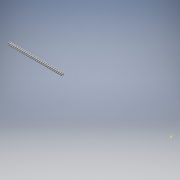
# Autodesk Inventor part: 40401m
Saved by Autodesk Inventor 2019 (Build 230136000, 136)
## iProperties
Company: TraceParts S.A.
Created: 2018-05-03
Part Number: 40401m
Checked By: TraceParts S.A.
Material: Aluminum 6061
Catalog Web Link: www.traceparts.com
Document SubType Name: Modeling
Designer: TraceParts
Density: 2.7 g/cm^3
Appearance: Aluminum - Dark
SUPPLIER_NAME: RS Components
SUPPLIER: Bosch Rexroth
RS_STOCK_NUMBER: 4597211
REVISION: A
DESIGN: Bosch Rexroth Aluminium Strut Profile, 10mm Groove , 3000mm L, 40 x 40mm strut profile
REFERENCE: 3842993120/3000
TIMESTAMP: 30/06/2015 16:02
TraceParts.PartVersion: 1.1.3
TraceParts.PartStatus: Published
TRACEPARTS: TRACEPARTS
TraceParts.InstanceId: 10-20072015-123890AZAWWE1HC2GQYC8QBJ8WTJ7U2
TraceParts.PartLanguage: en
TraceParts.PartTitle: Bosch Rexroth Aluminium Strut Profile, 10mm Groove , 3000mm L, 40 x 40mm strut profile
TraceParts.PartNumber: 10-20072015-123890
TraceParts.ClassPath: RS_COMPONENTS:10-20072015-123890
Author: TraceParts
Autodesk Inventor part; units mm, degrees
ref_plane "YZ Plane" through (0, 0, 0) normal (1, 0, 0) x (0, 1, 0)
ref_plane "XZ Plane" through (0, 0, 0) normal (0, 1, 0) x (-1, 0, 0)
ref_plane "XY Plane" through (0, 0, 0) normal (0, 0, 1) x (1, 0, 0)
ref_plane "Work Plane1" through (3000, -6.0858, -7.5) normal (1, 0, 0) x (0, 0, -1)
sketch "Sketch1" plane through (3000, -6.0858, -7.5) normal (1, 0, 0) x (0, 0, -1)
  line L0 (0, 0) -> (3.9642, -3.9642) projected
  line L1 (0, 12.1716) -> (0, 0) projected
  line L2 (3.9642, 16.1358) -> (0, 12.1716) projected
  line L3 (6.5, 16.1358) -> (3.9642, 16.1358) projected
  line L4 (6.5, 11.0858) -> (6.5, 16.1358) projected
  line L5 (11, 11.0858) -> (6.5, 11.0858) projected
  line L6 (11, 11.8858) -> (11, 11.0858) projected
  line L7 (12.5, 11.8858) -> (11, 11.8858) projected
  line L8 (12.5, 23.0858) -> (12.5, 11.8858) projected
  arc A0 (12.5, 23.0858) -> (9.5, 26.0858) centre (9.5, 23.0858) ccw projected
  line L9 (-1.7, 26.0858) -> (9.5, 26.0858) projected
  line L10 (-1.7, 24.5858) -> (-1.7, 26.0858) projected
  line L11 (-2.5, 24.5858) -> (-1.7, 24.5858) projected
  line L12 (-2.5, 20.0858) -> (-2.5, 24.5858) projected
  line L13 (2.55, 20.0858) -> (-2.5, 20.0858) projected
  line L14 (2.55, 17.55) -> (2.55, 20.0858) projected
  line L15 (-1.4142, 13.5858) -> (2.55, 17.55) projected
  line L16 (-13.5858, 13.5858) -> (-1.4142, 13.5858) projected
  line L17 (-17.55, 17.55) -> (-13.5858, 13.5858) projected
  line L18 (-17.55, 20.0858) -> (-17.55, 17.55) projected
  line L19 (-12.5, 20.0858) -> (-17.55, 20.0858) projected
  line L20 (-12.5, 24.5858) -> (-12.5, 20.0858) projected
  line L21 (-13.3, 24.5858) -> (-12.5, 24.5858) projected
  line L22 (-13.3, 26.0858) -> (-13.3, 24.5858) projected
  line L23 (-24.5, 26.0858) -> (-13.3, 26.0858) projected
  arc A1 (-24.5, 26.0858) -> (-27.5, 23.0858) centre (-24.5, 23.0858) ccw projected
  line L24 (-27.5, 11.8858) -> (-27.5, 23.0858) projected
  line L25 (-26, 11.8858) -> (-27.5, 11.8858) projected
  line L26 (-26, 11.0858) -> (-26, 11.8858) projected
  line L27 (-21.5, 11.0858) -> (-26, 11.0858) projected
  line L28 (-21.5, 16.1358) -> (-21.5, 11.0858) projected
  line L29 (-18.9642, 16.1358) -> (-21.5, 16.1358) projected
  line L30 (-15, 12.1716) -> (-18.9642, 16.1358) projected
  line L31 (-15, 0) -> (-15, 12.1716) projected
  line L32 (-18.9642, -3.9642) -> (-15, 0) projected
  line L33 (-21.5, -3.9642) -> (-18.9642, -3.9642) projected
  line L34 (-21.5, 1.0858) -> (-21.5, -3.9642) projected
  line L35 (-26, 1.0858) -> (-21.5, 1.0858) projected
  line L36 (-26, 0.2858) -> (-26, 1.0858) projected
  line L37 (-27.5, 0.2858) -> (-26, 0.2858) projected
  line L38 (-27.5, -10.9142) -> (-27.5, 0.2858) projected
  arc A2 (-27.5, -10.9142) -> (-24.5, -13.9142) centre (-24.5, -10.9142) ccw projected
  line L39 (-13.3, -13.9142) -> (-24.5, -13.9142) projected
  line L40 (-13.3, -12.4142) -> (-13.3, -13.9142) projected
  line L41 (-12.5, -12.4142) -> (-13.3, -12.4142) projected
  line L42 (-12.5, -7.9142) -> (-12.5, -12.4142) projected
  line L43 (-17.55, -7.9142) -> (-12.5, -7.9142) projected
  line L44 (-17.55, -5.3784) -> (-17.55, -7.9142) projected
  line L45 (-13.5858, -1.4142) -> (-17.55, -5.3784) projected
  line L46 (-1.4142, -1.4142) -> (-13.5858, -1.4142) projected
  line L47 (2.55, -5.3784) -> (-1.4142, -1.4142) projected
  line L48 (2.55, -7.9142) -> (2.55, -5.3784) projected
  line L49 (-2.5, -7.9142) -> (2.55, -7.9142) projected
  line L50 (-2.5, -12.4142) -> (-2.5, -7.9142) projected
  line L51 (-1.7, -12.4142) -> (-2.5, -12.4142) projected
  line L52 (-1.7, -13.9142) -> (-1.7, -12.4142) projected
  line L53 (9.5, -13.9142) -> (-1.7, -13.9142) projected
  arc A3 (9.5, -13.9142) -> (12.5, -10.9142) centre (9.5, -10.9142) ccw projected
  line L54 (12.5, 0.2858) -> (12.5, -10.9142) projected
  line L55 (11, 0.2858) -> (12.5, 0.2858) projected
  line L56 (11, 1.0858) -> (11, 0.2858) projected
  line L57 (6.5, 1.0858) -> (11, 1.0858) projected
  line L58 (6.5, -3.9642) -> (6.5, 1.0858) projected
  line L59 (3.9642, -3.9642) -> (6.5, -3.9642) projected
  line L60 (8, -1.9142) -> (11, -1.9142) projected
  line L61 (11, -1.9142) -> (11, -8.4142) projected
  line L62 (11, -8.4142) -> (9.75, -8.4142) projected
  arc A4 (7, -11.1642) -> (9.75, -8.4142) centre (7, -8.4142) ccw projected
  line L63 (7, -11.1642) -> (7, -12.4142) projected
  line L64 (7, -12.4142) -> (0.5, -12.4142) projected
  line L65 (0.5, -12.4142) -> (0.5, -9.4142) projected
  line L66 (0.5, -9.4142) -> (4.25, -9.4142) projected
  line L67 (4.25, -9.4142) -> (4.25, -8.4142) projected
  arc A5 (7, -5.6642) -> (4.25, -8.4142) centre (7, -8.4142) ccw projected
  line L68 (7, -5.6642) -> (8, -5.6642) projected
  line L69 (8, -5.6642) -> (8, -1.9142) projected
  line L70 (0.5, 21.5858) -> (0.5, 24.5858) projected
  line L71 (0.5, 24.5858) -> (7, 24.5858) projected
  line L72 (7, 24.5858) -> (7, 23.3358) projected
  arc A6 (9.75, 20.5858) -> (7, 23.3358) centre (7, 20.5858) ccw projected
  line L73 (9.75, 20.5858) -> (11, 20.5858) projected
  line L74 (11, 20.5858) -> (11, 14.0858) projected
  line L75 (11, 14.0858) -> (8, 14.0858) projected
  line L76 (8, 14.0858) -> (8, 17.8358) projected
  line L77 (8, 17.8358) -> (7, 17.8358) projected
  arc A7 (4.25, 20.5858) -> (7, 17.8358) centre (7, 20.5858) ccw projected
  line L78 (4.25, 20.5858) -> (4.25, 21.5858) projected
  line L79 (4.25, 21.5858) -> (0.5, 21.5858) projected
  line L80 (-23, 14.0858) -> (-26, 14.0858) projected
  line L81 (-26, 14.0858) -> (-26, 20.5858) projected
  line L82 (-26, 20.5858) -> (-24.75, 20.5858) projected
  arc A8 (-22, 23.3358) -> (-24.75, 20.5858) centre (-22, 20.5858) ccw projected
  line L83 (-22, 23.3358) -> (-22, 24.5858) projected
  line L84 (-22, 24.5858) -> (-15.5, 24.5858) projected
  line L85 (-15.5, 24.5858) -> (-15.5, 21.5858) projected
  line L86 (-15.5, 21.5858) -> (-19.25, 21.5858) projected
  line L87 (-19.25, 21.5858) -> (-19.25, 20.5858) projected
  arc A9 (-22, 17.8358) -> (-19.25, 20.5858) centre (-22, 20.5858) ccw projected
  line L88 (-22, 17.8358) -> (-23, 17.8358) projected
  line L89 (-23, 17.8358) -> (-23, 14.0858) projected
  line L90 (-15.5, -9.4142) -> (-15.5, -12.4142) projected
  line L91 (-15.5, -12.4142) -> (-22, -12.4142) projected
  line L92 (-22, -12.4142) -> (-22, -11.1642) projected
  arc A10 (-24.75, -8.4142) -> (-22, -11.1642) centre (-22, -8.4142) ccw projected
  line L93 (-24.75, -8.4142) -> (-26, -8.4142) projected
  line L94 (-26, -8.4142) -> (-26, -1.9142) projected
  line L95 (-26, -1.9142) -> (-23, -1.9142) projected
  line L96 (-23, -1.9142) -> (-23, -5.6642) projected
  line L97 (-23, -5.6642) -> (-22, -5.6642) projected
  arc A11 (-19.25, -8.4142) -> (-22, -5.6642) centre (-22, -8.4142) ccw projected
  line L98 (-19.25, -8.4142) -> (-19.25, -9.4142) projected
  line L99 (-19.25, -9.4142) -> (-15.5, -9.4142) projected
  line L100 (-9.4937, 1.5005) -> (-9.761, 0.8858) projected
  line L101 (-9.761, 0.8858) -> (-12.7, 0.8858) projected
  line L102 (-12.7, 0.8858) -> (-12.7, 3.8248) projected
  line L103 (-12.7, 3.8248) -> (-12.0853, 4.092) projected
  arc A12 (-12.0853, 8.0795) -> (-12.0853, 4.092) centre (-7.5, 6.0858) ccw projected
  line L104 (-12.0853, 8.0795) -> (-12.7, 8.3468) projected
  line L105 (-12.7, 8.3468) -> (-12.7, 11.2858) projected
  line L106 (-12.7, 11.2858) -> (-9.761, 11.2858) projected
  line L107 (-9.761, 11.2858) -> (-9.4937, 10.6711) projected
  arc A13 (-5.5063, 10.6711) -> (-9.4937, 10.6711) centre (-7.5, 6.0858) ccw projected
  line L108 (-5.5063, 10.6711) -> (-5.239, 11.2858) projected
  line L109 (-5.239, 11.2858) -> (-2.3, 11.2858) projected
  line L110 (-2.3, 11.2858) -> (-2.3, 8.3468) projected
  line L111 (-2.3, 8.3468) -> (-2.9147, 8.0795) projected
  arc A14 (-2.9147, 4.092) -> (-2.9147, 8.0795) centre (-7.5, 6.0858) ccw projected
  line L112 (-2.9147, 4.092) -> (-2.3, 3.8248) projected
  line L113 (-2.3, 3.8248) -> (-2.3, 0.8858) projected
  line L114 (-2.3, 0.8858) -> (-5.239, 0.8858) projected
  line L115 (-5.239, 0.8858) -> (-5.5063, 1.5005) projected
  arc A15 (-9.4937, 1.5005) -> (-5.5063, 1.5005) centre (-7.5, 6.0858) ccw projected
  point P0 (-7.5, 6.0858)
ref_plane "Work Plane2" through (0, -6.0858, -7.5) normal (-1, 0, 0) x (0, 0, 1)
sketch "Sketch2" plane through (0, -6.0858, -7.5) normal (-1, 0, 0) x (0, 0, 1)
  line L0 (0, 12.1716) -> (0, 0) projected
  line L1 (0, 0) -> (-3.9642, -3.9642) projected
  line L2 (-3.9642, -3.9642) -> (-6.5, -3.9642) projected
  line L3 (-6.5, -3.9642) -> (-6.5, 1.0858) projected
  line L4 (-6.5, 1.0858) -> (-11, 1.0858) projected
  line L5 (-11, 1.0858) -> (-11, 0.2858) projected
  line L6 (-11, 0.2858) -> (-12.5, 0.2858) projected
  line L7 (-12.5, 0.2858) -> (-12.5, -10.9142) projected
  arc A0 (-12.5, -10.9142) -> (-9.5, -13.9142) centre (-9.5, -10.9142) ccw projected
  line L8 (-9.5, -13.9142) -> (1.7, -13.9142) projected
  line L9 (1.7, -13.9142) -> (1.7, -12.4142) projected
  line L10 (1.7, -12.4142) -> (2.5, -12.4142) projected
  line L11 (2.5, -12.4142) -> (2.5, -7.9142) projected
  line L12 (2.5, -7.9142) -> (-2.55, -7.9142) projected
  line L13 (-2.55, -7.9142) -> (-2.55, -5.3784) projected
  line L14 (-2.55, -5.3784) -> (1.4142, -1.4142) projected
  line L15 (1.4142, -1.4142) -> (13.5858, -1.4142) projected
  line L16 (13.5858, -1.4142) -> (17.55, -5.3784) projected
  line L17 (17.55, -5.3784) -> (17.55, -7.9142) projected
  line L18 (17.55, -7.9142) -> (12.5, -7.9142) projected
  line L19 (12.5, -7.9142) -> (12.5, -12.4142) projected
  line L20 (12.5, -12.4142) -> (13.3, -12.4142) projected
  line L21 (13.3, -12.4142) -> (13.3, -13.9142) projected
  line L22 (13.3, -13.9142) -> (24.5, -13.9142) projected
  arc A1 (24.5, -13.9142) -> (27.5, -10.9142) centre (24.5, -10.9142) ccw projected
  line L23 (27.5, -10.9142) -> (27.5, 0.2858) projected
  line L24 (27.5, 0.2858) -> (26, 0.2858) projected
  line L25 (26, 0.2858) -> (26, 1.0858) projected
  line L26 (26, 1.0858) -> (21.5, 1.0858) projected
  line L27 (21.5, 1.0858) -> (21.5, -3.9642) projected
  line L28 (21.5, -3.9642) -> (18.9642, -3.9642) projected
  line L29 (18.9642, -3.9642) -> (15, 0) projected
  line L30 (15, 0) -> (15, 12.1716) projected
  line L31 (15, 12.1716) -> (18.9642, 16.1358) projected
  line L32 (18.9642, 16.1358) -> (21.5, 16.1358) projected
  line L33 (21.5, 16.1358) -> (21.5, 11.0858) projected
  line L34 (21.5, 11.0858) -> (26, 11.0858) projected
  line L35 (26, 11.0858) -> (26, 11.8858) projected
  line L36 (26, 11.8858) -> (27.5, 11.8858) projected
  line L37 (27.5, 11.8858) -> (27.5, 23.0858) projected
  arc A2 (27.5, 23.0858) -> (24.5, 26.0858) centre (24.5, 23.0858) ccw projected
  line L38 (24.5, 26.0858) -> (13.3, 26.0858) projected
  line L39 (13.3, 26.0858) -> (13.3, 24.5858) projected
  line L40 (13.3, 24.5858) -> (12.5, 24.5858) projected
  line L41 (12.5, 24.5858) -> (12.5, 20.0858) projected
  line L42 (12.5, 20.0858) -> (17.55, 20.0858) projected
  line L43 (17.55, 20.0858) -> (17.55, 17.55) projected
  line L44 (17.55, 17.55) -> (13.5858, 13.5858) projected
  line L45 (13.5858, 13.5858) -> (1.4142, 13.5858) projected
  line L46 (1.4142, 13.5858) -> (-2.55, 17.55) projected
  line L47 (-2.55, 17.55) -> (-2.55, 20.0858) projected
  line L48 (-2.55, 20.0858) -> (2.5, 20.0858) projected
  line L49 (2.5, 20.0858) -> (2.5, 24.5858) projected
  line L50 (2.5, 24.5858) -> (1.7, 24.5858) projected
  line L51 (1.7, 24.5858) -> (1.7, 26.0858) projected
  line L52 (1.7, 26.0858) -> (-9.5, 26.0858) projected
  arc A3 (-9.5, 26.0858) -> (-12.5, 23.0858) centre (-9.5, 23.0858) ccw projected
  line L53 (-12.5, 23.0858) -> (-12.5, 11.8858) projected
  line L54 (-12.5, 11.8858) -> (-11, 11.8858) projected
  line L55 (-11, 11.8858) -> (-11, 11.0858) projected
  line L56 (-11, 11.0858) -> (-6.5, 11.0858) projected
  line L57 (-6.5, 11.0858) -> (-6.5, 16.1358) projected
  line L58 (-6.5, 16.1358) -> (-3.9642, 16.1358) projected
  line L59 (-3.9642, 16.1358) -> (0, 12.1716) projected
  line L60 (-11, -1.9142) -> (-8, -1.9142) projected
  line L61 (-8, -1.9142) -> (-8, -5.6642) projected
  line L62 (-8, -5.6642) -> (-7, -5.6642) projected
  arc A4 (-4.25, -8.4142) -> (-7, -5.6642) centre (-7, -8.4142) ccw projected
  line L63 (-4.25, -8.4142) -> (-4.25, -9.4142) projected
  line L64 (-4.25, -9.4142) -> (-0.5, -9.4142) projected
  line L65 (-0.5, -9.4142) -> (-0.5, -12.4142) projected
  line L66 (-0.5, -12.4142) -> (-7, -12.4142) projected
  line L67 (-7, -12.4142) -> (-7, -11.1642) projected
  arc A5 (-9.75, -8.4142) -> (-7, -11.1642) centre (-7, -8.4142) ccw projected
  line L68 (-9.75, -8.4142) -> (-11, -8.4142) projected
  line L69 (-11, -8.4142) -> (-11, -1.9142) projected
  line L70 (-0.5, 24.5858) -> (-0.5, 21.5858) projected
  line L71 (-0.5, 21.5858) -> (-4.25, 21.5858) projected
  line L72 (-4.25, 21.5858) -> (-4.25, 20.5858) projected
  arc A6 (-7, 17.8358) -> (-4.25, 20.5858) centre (-7, 20.5858) ccw projected
  line L73 (-7, 17.8358) -> (-8, 17.8358) projected
  line L74 (-8, 17.8358) -> (-8, 14.0858) projected
  line L75 (-8, 14.0858) -> (-11, 14.0858) projected
  line L76 (-11, 14.0858) -> (-11, 20.5858) projected
  line L77 (-11, 20.5858) -> (-9.75, 20.5858) projected
  arc A7 (-7, 23.3358) -> (-9.75, 20.5858) centre (-7, 20.5858) ccw projected
  line L78 (-7, 23.3358) -> (-7, 24.5858) projected
  line L79 (-7, 24.5858) -> (-0.5, 24.5858) projected
  line L80 (26, 14.0858) -> (23, 14.0858) projected
  line L81 (23, 14.0858) -> (23, 17.8358) projected
  line L82 (23, 17.8358) -> (22, 17.8358) projected
  arc A8 (19.25, 20.5858) -> (22, 17.8358) centre (22, 20.5858) ccw projected
  line L83 (19.25, 20.5858) -> (19.25, 21.5858) projected
  line L84 (19.25, 21.5858) -> (15.5, 21.5858) projected
  line L85 (15.5, 21.5858) -> (15.5, 24.5858) projected
  line L86 (15.5, 24.5858) -> (22, 24.5858) projected
  line L87 (22, 24.5858) -> (22, 23.3358) projected
  arc A9 (24.75, 20.5858) -> (22, 23.3358) centre (22, 20.5858) ccw projected
  line L88 (24.75, 20.5858) -> (26, 20.5858) projected
  line L89 (26, 20.5858) -> (26, 14.0858) projected
  line L90 (15.5, -12.4142) -> (15.5, -9.4142) projected
  line L91 (15.5, -9.4142) -> (19.25, -9.4142) projected
  line L92 (19.25, -9.4142) -> (19.25, -8.4142) projected
  arc A10 (22, -5.6642) -> (19.25, -8.4142) centre (22, -8.4142) ccw projected
  line L93 (22, -5.6642) -> (23, -5.6642) projected
  line L94 (23, -5.6642) -> (23, -1.9142) projected
  line L95 (23, -1.9142) -> (26, -1.9142) projected
  line L96 (26, -1.9142) -> (26, -8.4142) projected
  line L97 (26, -8.4142) -> (24.75, -8.4142) projected
  arc A11 (22, -11.1642) -> (24.75, -8.4142) centre (22, -8.4142) ccw projected
  line L98 (22, -11.1642) -> (22, -12.4142) projected
  line L99 (22, -12.4142) -> (15.5, -12.4142) projected
  line L100 (9.761, 0.8858) -> (9.4937, 1.5005) projected
  arc A12 (5.5063, 1.5005) -> (9.4937, 1.5005) centre (7.5, 6.0858) ccw projected
  line L101 (5.5063, 1.5005) -> (5.239, 0.8858) projected
  line L102 (5.239, 0.8858) -> (2.3, 0.8858) projected
  line L103 (2.3, 0.8858) -> (2.3, 3.8248) projected
  line L104 (2.3, 3.8248) -> (2.9147, 4.092) projected
  arc A13 (2.9147, 8.0795) -> (2.9147, 4.092) centre (7.5, 6.0858) ccw projected
  line L105 (2.9147, 8.0795) -> (2.3, 8.3468) projected
  line L106 (2.3, 8.3468) -> (2.3, 11.2858) projected
  line L107 (2.3, 11.2858) -> (5.239, 11.2858) projected
  line L108 (5.239, 11.2858) -> (5.5063, 10.6711) projected
  arc A14 (9.4937, 10.6711) -> (5.5063, 10.6711) centre (7.5, 6.0858) ccw projected
  line L109 (9.4937, 10.6711) -> (9.761, 11.2858) projected
  line L110 (9.761, 11.2858) -> (12.7, 11.2858) projected
  line L111 (12.7, 11.2858) -> (12.7, 8.3468) projected
  line L112 (12.7, 8.3468) -> (12.0853, 8.0795) projected
  arc A15 (12.0853, 4.092) -> (12.0853, 8.0795) centre (7.5, 6.0858) ccw projected
  line L113 (12.0853, 4.092) -> (12.7, 3.8248) projected
  line L114 (12.7, 3.8248) -> (12.7, 0.8858) projected
  line L115 (12.7, 0.8858) -> (9.761, 0.8858) projected
  point P0 (7.5, 6.0858)
extrude "Extrusion2" add sketch "Sketch2" against normal blind 1000
body "Solid2"
